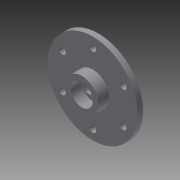
# Autodesk Inventor part: MotorHub
Saved by Autodesk Inventor 2014 (Build 180170000, 170)
## iProperties
Created: 2014-03-25
Part Number: MotorHub
Material: Generic
Document SubType Name: Modeling
Designer: Lauszus
Density: 1 g/cm^3
Appearance: Default
Author: Lauszus
Autodesk Inventor part; units mm, degrees
ref_plane "YZ Plane" through (0, 0, 0) normal (1, 0, 0) x (0, 1, 0)
ref_plane "XZ Plane" through (0, 0, 0) normal (0, 1, 0) x (-1, 0, 0)
ref_plane "XY Plane" through (0, 0, 0) normal (0, 0, 1) x (1, 0, 0)
sketch "Sketch1" plane through (0, 0, 0) normal (0, 1, 0) x (-1, 0, 0)
  circle A0 centre (0, 0) radius 41
  circle A1 centre (-0.0062, 32) radius 3.05
  circle A2 centre (0.0062, -32) radius 3.05
  circle A3 centre (27.7097, 16.0054) radius 3.05
  circle A4 centre (27.7159, -15.9946) radius 3.05
  circle A5 centre (-27.7097, -16.0054) radius 3.05
  circle A6 centre (-27.7159, 15.9946) radius 3.05
  line L0 (-6.0019, -5.8408) -> (6.0022, 5.8411) construction
  line L1 (0, 0) -> (0, 0)
  line L2 (0, -6) -> (6.1612, -6)
  line L3 (-6.1612, 6) -> (0, 6)
  line L4 (6.1612, -6) -> (-6.1612, -6)
  line L5 (-6.1612, 6) -> (6.1612, 6)
  arc A7 (6.1612, -6) -> (6.1612, 6) centre (0, 0) ccw
  arc A8 (-6.1612, 6) -> (-6.1612, -6) centre (0, 0) ccw
  dimension "d0" = 82
  dimension "d6" = 6.1
  dimension "d32" = 12
  dimension "d34" = 17.2
  dimension "d35" = 60
  dimension "d36" = 32
  dimension "d37" = 32
  dimension "d38" = 60
  dimension "d39" = 60
  dimension "d40" = 60
  dimension "d41" = 60
  dimension "d43" = 32
  dimension "d44" = 32
  dimension "d45" = 32
  dimension "d46" = 32
  dimension "d47" = 60
  dimension "d50" = 6.1
  dimension "d51" = 6.1
  dimension "d52" = 6.1
  dimension "d53" = 6.1
  dimension "d54" = 6.1
  constraints: 12 end point, 9 centre point, 4 point on circle, 2 coincident, 1 parallel, 1 point on line, 1 vertical
  measures "d0" diameter of A0
  measures "d6" diameter of A2
  measures "d32" distance of L2.start L3.end
  measures "d34" distance of L3.start L2.end
  measures "d36" distance of A1.centre L1.end
  measures "d37" distance of A2.centre A0.centre
  measures "d43" distance of A3.centre A0.centre
  measures "d44" distance of A5.centre point (0, 0)
  measures "d45" distance of A6.centre L1.end
  measures "d46" distance of A4.centre L1.end
  measures "d50" diameter of A1
  measures "d51" diameter of A6
  measures "d52" diameter of A5
  measures "d53" diameter of A4
  measures "d54" diameter of A3
extrude "Extrusion3" add sketch "Sketch1" along normal blind 5
sketch "Sketch2" plane through (0, 0, 0) normal (0, -1, 0) x (1, 0, 0)
  circle A0 centre (0, 0) radius 41 projected
  circle A1 centre (0, 0) radius 10
  circle A2 centre (0, 0) radius 15
  dimension "d55" = 20
  dimension "d56" = 30
  constraints: 2 centre point, 2 coincident
  measures "d55" diameter of A1
  measures "d56" diameter of A2
extrude "Extrusion4" add sketch "Sketch2" along normal blind 10 contours A2
body "Solid3"
